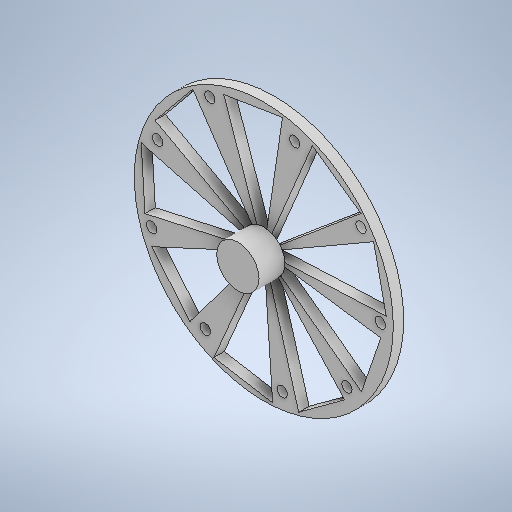
# Autodesk Inventor part: F 3
Saved by Autodesk Inventor 2025.1 (Build 291241000, 241)
## iProperties
Created: 2025-04-19
Part Number: F 3
Material: Generic
Document SubType Name: Modeling
Designer: POORNIMA HIREMATH
Density: 1 g/cm^3
Appearance: Default
Author: POORNIMA HIREMATH
Autodesk Inventor part; units mm, degrees
ref_plane "YZ Plane" through (0, 0, 0) normal (1, 0, 0) x (0, 1, 0)
ref_plane "XZ Plane" through (0, 0, 0) normal (0, 1, 0) x (-1, 0, 0)
ref_plane "XY Plane" through (0, 0, 0) normal (0, 0, 1) x (1, 0, 0)
sketch "Sketch1" plane through (0, 0, 0) normal (0, 0, 1) x (1, 0, 0)
  circle A0 centre (0, 0) radius 25
  dimension "d0" = 50
  constraints: 1 centre point, 1 coincident
  measures "d0" diameter of A0
extrude "Extrusion1" add sketch "Sketch1" along normal blind 2
sketch "Sketch2" plane through (0, 0, 2) normal (0, 0, 1) x (1, 0, 0)
  line L0 (0, 0) -> (21.2176, 12.25)
  line L1 (0, 0) -> (24.5, 0) construction
  line L2 (21.2176, 12.25) -> (23.6504, 1.0103)
  circle A0 centre (0, 0) radius 25 projected
  line L3 (23.6504, 1.0103) -> (0, 0)
  dimension "d3" = 24.5
  dimension "d4" = 30
  dimension "d5" = 11.5
  constraints: 8 end point, 1 equal length, 1 horizontal
  measures "d3" distance of L0.start L0.end
  measures "d4" angle of L1 L0
  measures "d5" distance of L0.end L2.end
extrude "Extrusion2" cut sketch "Sketch2" against normal blind 2 contours L0 L2 L3
sketch "Sketch3" plane through (0, 0, 2) normal (0, 0, 1) x (1, 0, 0)
  point P0 (0, 0)
sketch "Sketch4" plane through (0, 0, 2) normal (0, 0, 1) x (1, 0, 0)
  line L0 (0, 0) -> (23.6504, 1.0103) projected
  line L1 (0, 0) -> (18.7681, 15.7483)
  line L2 (0, 0) -> (24.5, 0) construction
  line L3 (18.7681, 15.7483) -> (9.384, 22.3958)
  line L4 (9.384, 22.3958) -> (0, 0)
  dimension "d8" = 24.5
  dimension "d9" = 40
  dimension "d10" = 11.5
  constraints: 8 end point, 1 equal length, 1 horizontal
  measures "d8" distance of L0.start L1.end
  measures "d9" angle of L2 L1
  measures "d10" distance of L1.end L3.end
extrude "Extrusion3" cut sketch "Sketch4" against normal blind 2
sketch "Sketch5" plane through (0, 0, 2) normal (0, 0, 1) x (1, 0, 0)
  line L0 (23.6504, 1.0103) -> (0, 0) projected
  line L1 (0, 0) -> (3.6213, 24.2309)
  line L2 (0, 0) -> (24.5, 0) construction
  line L3 (3.6213, 24.2309) -> (-7.7313, 22.3958)
  line L4 (9.384, 22.3958) -> (0, 0) projected
  line L5 (-7.7313, 22.3958) -> (0, 0)
  dimension "d13" = 24.5
  dimension "d14" = 81.5
  dimension "d15" = 11.5
  constraints: 8 end point, 1 equal length, 1 horizontal
  measures "d13" distance of L0.end L1.end
  measures "d14" angle of L2 L1
  measures "d15" distance of L1.end L3.end
extrude "Extrusion4" cut sketch "Sketch5" against normal blind 2
sketch "Sketch6" plane through (0, 0, 2) normal (0, 0, 1) x (1, 0, 0)
  line L0 (0, 0) -> (-13.7002, 20.3114)
  line L1 (0, 0) -> (24.5, 0) construction
  line L2 (-13.7002, 20.3114) -> (-20.9994, 11.4248)
  circle A0 centre (0, 0) radius 25 projected
  line L3 (-20.9994, 11.4248) -> (0, 0)
  dimension "d18" = 24.5
  dimension "d19" = 124
  dimension "d20" = 11.5
  constraints: 8 end point, 1 equal length, 1 horizontal
  measures "d18" distance of L0.start L0.end
  measures "d19" angle of L1 L0
  measures "d20" distance of L0.end L2.end
extrude "Extrusion5" cut sketch "Sketch6" against normal blind 2 contours L3 L2 L0
sketch "Sketch7" plane through (0, 0, 2) normal (0, 0, 1) x (1, 0, 0)
  line L0 (23.6504, 1.0103) -> (0, 0) projected
  line L1 (0, 0) -> (-23.6652, 6.3411)
  line L2 (0, 0) -> (24.5, 0) construction
  line L3 (-23.6652, 6.3411) -> (-22.9423, -5.1362)
  circle A0 centre (0, 0) radius 25 projected
  line L4 (-22.9423, -5.1362) -> (0, 0)
  dimension "d23" = 24.5
  dimension "d24" = 165
  dimension "d25" = 11.5
  constraints: 8 end point, 1 equal length, 1 horizontal
  measures "d23" distance of L0.end L1.end
  measures "d24" angle of L2 L1
  measures "d25" distance of L1.end L3.end
extrude "Extrusion6" cut sketch "Sketch7" against normal blind 2 contours L4 L3 L1
sketch "Sketch8" plane through (0, 0, 2) normal (0, 0, 1) x (1, 0, 0)
  line L0 (0, 0) -> (-21.6423, -10.0067)
  line L1 (-21.6423, -10.0067) -> (-14.2585, -18.8231)
  line L2 (-14.2585, -18.8231) -> (0, 0)
  dimension "d28" = 11.5
  constraints: 6 end point, 1 point on line
  measures "d28" distance of L0.end L1.end
extrude "Extrusion7" cut sketch "Sketch8" against normal blind 2
sketch "Sketch9" plane through (0, 0, 2) normal (0, 0, 1) x (1, 0, 0)
  line L0 (0, 0) -> (-21.6423, -10.0067) projected
  line L1 (0, 0) -> (-9.6274, -22.5292)
  line L2 (-9.6274, -22.5292) -> (1.7119, -24.4448)
  line L3 (1.7119, -24.4448) -> (0, 0)
  dimension "d31" = 24.5
  dimension "d32" = 11.5
  constraints: 6 end point
  measures "d31" distance of L0.start L1.end
  measures "d32" distance of L1.end L2.end
extrude "Extrusion8" cut sketch "Sketch9" against normal blind 2
sketch "Sketch10" plane through (0, 0, 2) normal (0, 0, 1) x (1, 0, 0)
  line L0 (0, 0) -> (6.7487, -23.5)
  line L1 (6.7487, -23.5) -> (15.6191, -16.995)
  line L2 (15.6191, -16.995) -> (0, 0)
  dimension "d35" = 11
  dimension "d36" = 23.5
  constraints: 6 end point
  measures "d35" distance of L0.end L1.end
  measures "d36" vertical distance of L0.start L0.end
extrude "Extrusion9" cut sketch "Sketch10" against normal blind 2
sketch "Sketch11" plane through (0, 0, 2) normal (0, 0, 1) x (1, 0, 0)
  line L0 (0, 0) -> (-22.9423, -5.1362) projected
  line L1 (0, 0) -> (18.8673, -14.0098)
  line L2 (18.8673, -14.0098) -> (22.6101, -3.1358)
  line L3 (0, 0) -> (23.6504, 1.0103) projected
  line L4 (22.6101, -3.1358) -> (0, 0)
  dimension "d39" = 23.5
  dimension "d40" = 11.5
  constraints: 6 end point
  measures "d39" distance of L0.start L1.end
  measures "d40" distance of L1.end L2.end
extrude "Extrusion10" cut sketch "Sketch11" against normal blind 2
sketch "Sketch12" plane through (0, 0, 2) normal (0, 0, 1) x (1, 0, 0)
  line L0 (-21.6423, -10.0067) -> (0, 0) projected
  circle A0 centre (0, 0) radius 1.5
  dimension "d43" = 3
  constraints: 1 centre point, 1 coincident
  measures "d43" diameter of A0
extrude "Extrusion11" cut sketch "Sketch12" against normal blind 2
sketch "Sketch13" plane through (0, 0, 2) normal (0, 0, 1) x (1, 0, 0)
  circle A0 centre (-10.4058, 20.5939) radius 1
  point P0 (0, 0)
  dimension "d46" = 2
  constraints: 1 centre point
  measures "d46" diameter of A0
extrude "Extrusion12" cut sketch "Sketch13" against normal blind 2
sketch "Sketch14" plane through (0, 0, 2) normal (0, 0, 1) x (1, 0, 0)
  circle A0 centre (5.9648, 21.3776) radius 1
  point P0 (0, 0)
  dimension "d49" = 2
  constraints: 1 centre point
  measures "d49" diameter of A0
extrude "Extrusion13" cut sketch "Sketch14" against normal blind 2
sketch "Sketch15" plane through (0, 0, 2) normal (0, 0, 1) x (1, 0, 0)
  circle A0 centre (18.7681, 13.4535) radius 1
  point P0 (0, 0)
  dimension "d52" = 2
  constraints: 1 centre point
  measures "d52" diameter of A0
extrude "Extrusion14" cut sketch "Sketch15" against normal blind 2
sketch "Sketch16" plane through (0, 0, 2) normal (0, 0, 1) x (1, 0, 0)
  circle A0 centre (22.5096, -0.6531) radius 1
  point P0 (0, 0)
  dimension "d55" = 2
  constraints: 1 centre point
  measures "d55" diameter of A0
extrude "Extrusion15" cut sketch "Sketch16" against normal blind 2
sketch "Sketch17" plane through (0, 0, 2) normal (0, 0, 1) x (1, 0, 0)
  circle A0 centre (16.0659, -14.5855) radius 1
  point P0 (0, 0)
  dimension "d58" = 2
  constraints: 1 centre point
  measures "d58" diameter of A0
extrude "Extrusion16" cut sketch "Sketch17" against normal blind 2
sketch "Sketch18" plane through (0, 0, 2) normal (0, 0, 1) x (1, 0, 0)
  circle A0 centre (3.5814, -21.6389) radius 1
  point P0 (0, 0)
  dimension "d61" = 2
  constraints: 1 centre point
  measures "d61" diameter of A0
extrude "Extrusion17" cut sketch "Sketch18" against normal blind 2
sketch "Sketch19" plane through (0, 0, 2) normal (0, 0, 1) x (1, 0, 0)
  circle A0 centre (-11.2766, -18.5911) radius 1
  point P0 (0, 0)
  dimension "d64" = 2
  constraints: 1 centre point
  measures "d64" diameter of A0
extrude "Extrusion18" cut sketch "Sketch19" against normal blind 2
sketch "Sketch20" plane through (0, 0, 2) normal (0, 0, 1) x (1, 0, 0)
  circle A0 centre (-21.6423, -6.7485) radius 1
  point P0 (0, 0)
  dimension "d67" = 2
  constraints: 1 centre point
  measures "d67" diameter of A0
extrude "Extrusion19" cut sketch "Sketch20" against normal blind 2
sketch "Sketch21" plane through (0, 0, 2) normal (0, 0, 1) x (1, 0, 0)
  circle A0 centre (-20.5068, 8.403) radius 1
  point P0 (0, 0)
  dimension "d70" = 2
  constraints: 1 centre point
  measures "d70" diameter of A0
extrude "Extrusion20" cut sketch "Sketch21" against normal blind 2
sketch "Sketch22" plane through (0, 0, 2) normal (0, 0, 1) x (1, 0, 0)
  circle A0 centre (0, 0) radius 4.0832
  constraints: 1 centre point, 1 coincident
extrude "Extrusion21" add sketch "Sketch22" along normal blind 5
body "Solid1"
